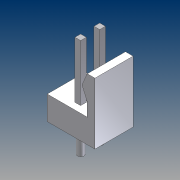
# Autodesk Inventor part: Molex KK 2 Pin
Saved by Autodesk Inventor 2012 (Build 160160000, 160)
## iProperties
Company: Team 801
Created: 2007-11-01
Part Number: Molex KK 2 Pin
Document SubType Name: Modeling
Designer: Jeffrey M
Manufacturer: Standard
Standards Organization: Custom
Mass: 0.146261 g
Surface Area: 2.63206 cm^2
Volume: 0.146261 cm^3
Density: 1 g/cm^3
Catalog Web Link: www.team801.org
Material: Default
PartAngTol0: 0.50 deg
PartAngTol1: 0.50 deg
PartAngTol2: 0.50 deg
PartLinTol0: 0.01 in
PartLinTol1: 0.01 in
PartLinTol2: 0.01 in
PartLinTol3: 0.005 in
PartAngTol3: 0deg30'
Author: Jeffrey M
Autodesk Inventor part; units mm, degrees
ref_plane "YZ Plane (RIGHT)" through (0, 0, 0) normal (1, 0, 0) x (0, 1, 0)
ref_plane "XZ Plane (TOP)" through (0, 0, 0) normal (0, 1, 0) x (-1, 0, 0)
ref_plane "XY Plane (FRONT)" through (0, 0, 0) normal (0, 0, 1) x (1, 0, 0)
sketch "Sketch2" plane through (0, 0, 0) normal (0, 0, 1) x (1, 0, 0)
  line L0 (-4.445, 0) -> (4.445, 0) construction
  line L1 (0, 9.8146) -> (0, -1.6358) construction
  line L2 (-3.175, 0) -> (3.175, 0)
  line L3 (2.159, 3.175) -> (-3.175, 3.175)
  line L4 (-3.175, 3.175) -> (-3.175, 0)
  line L5 (3.175, 0) -> (3.175, 8.1788)
  line L6 (3.175, 8.1788) -> (2.159, 8.1788)
  line L7 (2.159, 8.1788) -> (1.4478, 6.5607)
  line L8 (1.4478, 6.5607) -> (2.159, 4.9425)
  line L9 (2.159, 4.9425) -> (2.159, 3.175)
  point P0 (0, 0)
  dimension "d0" = 6.35
  dimension "d1" = 3.175
  dimension "d2" = 8.1788
  dimension "d3" = 1.4478
  dimension "d4" = 1.016
  constraints: 16 end point, 3 parallel, 2 equal length, 2 perpendicular, 2 point on line, 1 horizontal, 1 other
  measures "d0" distance of L2.start L2.end
  measures "d1" distance of L3.end L2.start
  measures "d2" distance of L2.end L5.end
  measures "d3" distance from line of L1 L7.end
  measures "d4" distance between parallel lines of L5 L9
extrude "Extrusion1" add sketch "Sketch2" along normal mid plane 2.54
sketch "Sketch3" plane through (-3.175, 0, 1.27) normal (0, -1, 0) x (1, 0, 0)
  line L0 (-1.27, -1.27) -> (7.62, -1.27) construction
  line L1 (3.175, 0.508) -> (3.175, -3.048) construction
  line L2 (2.794, -0.889) -> (3.556, -0.889)
  line L3 (3.556, -0.889) -> (3.556, -1.651)
  line L4 (3.556, -1.651) -> (2.794, -1.651)
  line L5 (2.794, -1.651) -> (2.794, -0.889)
  circle A0 centre (3.175, -1.27) radius 0.4445
  dimension "d7" = 0.762
  dimension "d15" = 0.889
  constraints: 8 end point, 2 parallel, 2 perpendicular, 1 centre point, 1 coincident, 1 horizontal, 2 other
  measures "d7" distance of L2.start L2.end
  measures "d15" diameter of A0
extrude "Extrusion2" add sketch "Sketch3" along normal blind 2.794 contours A0 L2 | L2 A0 L3 L4 L5 | L5 A0 | A0 L3 | L4 A0
extrude "Extrusion3" add sketch "Sketch3" against normal blind 10.668 contours L2 A0 L5 | L2 A0 L3 L4 L5 | L2 L3 A0 | A0 L4 L5 | L3 L4 A0
pattern_linear "Rectangular Pattern1" count 2 spacing 2.54 along (0, 0, 1) of "Extrusion1", "Extrusion2", "Extrusion3"
body "Solid1"
